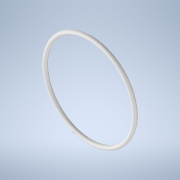
# Autodesk Inventor part: O-Ring_53_2_5
Saved by Autodesk Inventor 2022 (Build 260153000, 153)
## iProperties
Created: 2020-11-13
Part Number: O-Ring_53_2_5
Material: Generisch
Document SubType Name: Modeling
Designer: g.schardt
Density: 1 g/cm^3
Appearance: Vorgabe
Author: g.schardt
Autodesk Inventor part; units mm, degrees
ref_plane "YZ Plane" through (0, 0, 0) normal (1, 0, 0) x (0, 1, 0)
ref_plane "XZ Plane" through (0, 0, 0) normal (0, 1, 0) x (-1, 0, 0)
ref_plane "XY Plane" through (0, 0, 0) normal (0, 0, 1) x (1, 0, 0)
sketch "Skizze1" plane through (0, 0, 0) normal (1, 0, 0) x (0, 1, 0)
  circle A0 centre (-27.75, 0) radius 1.25
  line L0 (0, -1.75) -> (0, 1.75) projected
  point P0 (0, 0)
  dimension "d5" = 27.75
  constraints: 1 centre point, 1 horizontal alignment, 1 other
  measures "d5" distance of A0.centre point (0, 0)
revolve "Umdrehung1" add sketch "Skizze1" angle 360 about axis through (0, 0, -10) along (0, 0, 1)
